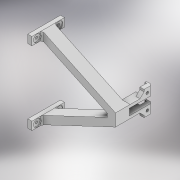
# Autodesk Inventor part: LickModule_temp
Saved by Autodesk Inventor 2020 (Build 240168000, 168)
## iProperties
Created: 2020-01-13
Part Number: LickModule_temp
Material: 일반
Document SubType Name: Modeling
Designer: Knowblesse
Density: 1 g/cm^3
Appearance: 기본값
Author: Knowblesse
## iProperties of the stored document _3D 인쇄.ipt
Created: 2021-10-22
Part Number: _3D 인쇄
Material: 일반
Document SubType Name: Modeling
Designer: Knowblesse
Density: 1 g/cm^3
Appearance: 기본값
Author: Knowblesse
Autodesk Inventor part; units mm, degrees
ref_plane "YZ Plane" through (0, 0, 0) normal (1, 0, 0) x (0, 1, 0)
ref_plane "XZ Plane" through (0, 0, 0) normal (0, 1, 0) x (-1, 0, 0)
ref_plane "XY Plane" through (0, 0, 0) normal (0, 0, 1) x (1, 0, 0)
sketch "스케치1" plane through (0, 0, 0) normal (0, 0, 1) x (1, 0, 0)
  line L0 (0, -40) -> (0, -50)
  line L1 (0, -50) -> (90, -7.5)
  line L2 (90, -7.5) -> (90, 7.5)
  line L3 (90, 7.5) -> (0, 50)
  line L4 (0, 50) -> (0, 40)
  line L5 (0, 40) -> (80, 2.2222)
  line L6 (80, 2.2222) -> (80, -2.2222)
  line L7 (80, -2.2222) -> (0, -40)
  point P0 (0, 0)
  point P1 (80, 0)
  point P2 (90, 0)
  point P3 (0, 45)
  dimension "d0" = 10
  dimension "d1" = 10
  dimension "d3" = 10
  dimension "d4" = 80
  dimension "d7" = 15
  dimension "d24" = 90
  constraints: 16 end point, 4 parallel, 3 midpoint, 2 horizontal alignment, 2 point on line, 1 vertical, 1 vertical alignment
  measures "d0" distance of L0.start L0.end
  measures "d1" distance of L3.end L4.end
  measures "d3" distance between parallel lines of L6 L2
  measures "d4" distance of L0.start L4.end
  measures "d7" distance of L1.end L2.end
  measures "d24" distance from line of point (0, 0) L2
extrude "돌출1" add sketch "스케치1" along normal blind 15
sketch "스케치2" plane through (0, 0, 0) normal (0, 0, -1) x (-1, 0, 0)
  line L0 (0, 40) -> (-80, 2.2222) projected
  line L1 (0, 50) -> (0, 40) projected
  line L2 (-90, 7.5) -> (0, 50) projected
  line L3 (-90, -7.5) -> (-90, 7.5) projected
  line L4 (0, -50) -> (-90, -7.5) projected
  line L5 (0, -40) -> (0, -50) projected
  line L6 (-80, -2.2222) -> (0, -40) projected
  line L7 (-80, 2.2222) -> (-80, -2.2222) projected
  line L8 (-90, -7.5) -> (-80, -7.5)
  line L9 (-80, -7.5) -> (-80, 7.5)
  line L10 (-80, 7.5) -> (-90, 7.5)
  line L11 (-90, 7.5) -> (-90, -7.5)
  line L12 (-80, 2.2222) -> (-80, -2.2222) projected
  point P0 (0, 0)
  point P1 (-85, 7.5)
  point P2 (-80, -2.2222)
  point P3 (-80, 2.2222)
  constraints: 8 end point, 2 parallel, 1 collinear, 1 horizontal, 1 horizontal alignment, 1 midpoint, 1 perpendicular
extrude "돌출2" add sketch "스케치2" along normal blind 30 contours L7 L9 L8 L3 L10
sketch "스케치3" plane through (0, -50, 0) normal (-1, 0, 0) x (0, 0, 1)
  line L0 (0, 100) -> (0, 90) projected
  line L1 (0, 90) -> (15, 90) projected
  line L2 (15, 100) -> (15, 90) projected
  line L3 (0, 100) -> (15, 100) projected
  line L4 (0, 10) -> (0, 0) projected
  line L5 (0, 0) -> (15, 0) projected
  line L6 (15, 10) -> (15, 0) projected
  line L7 (0, 10) -> (15, 10) projected
  line L8 (27.5, 100) -> (-12.5, 100)
  line L9 (-12.5, 100) -> (-12.5, 90)
  line L10 (-12.5, 90) -> (27.5, 90)
  line L11 (27.5, 90) -> (27.5, 100)
  line L12 (27.5, 10) -> (-12.5, 10)
  line L13 (-12.5, 10) -> (-12.5, 0)
  line L14 (-12.5, 0) -> (27.5, 0)
  line L15 (27.5, 0) -> (27.5, 10)
  line L16 (0, 90) -> (15, 90) projected
  line L17 (0, 0) -> (15, 0) projected
  line L18 (0, 10) -> (15, 10) projected
  line L19 (0, 100) -> (15, 100) projected
  point P0 (0, 50)
  point P1 (7.5, 10)
  point P2 (0, 10)
  point P3 (15, 10)
  point P4 (15, 0)
  dimension "d12" = 40
  constraints: 16 end point, 5 collinear, 4 parallel, 2 horizontal, 2 midpoint, 2 perpendicular, 1 point on line
  measures "d12" distance of L8.start L8.end
extrude "돌출3" add sketch "스케치3" along normal blind 5
sketch "스케치5" plane through (0, -50, 0) normal (1, 0, 0) x (0, 0, -1)
  line L0 (-27.5, 0) -> (-27.5, 10) projected
  line L1 (-27.5, 10) -> (12.5, 10) projected
  line L2 (12.5, 10) -> (12.5, 0) projected
  line L3 (-27.5, 90) -> (-27.5, 100) projected
  line L4 (-27.5, 100) -> (12.5, 100) projected
  line L5 (12.5, 100) -> (12.5, 90) projected
  line L6 (12.5, 90) -> (-27.5, 90) projected
  line L7 (12.5, 0) -> (-27.5, 0) projected
  point P0 (0, 50)
  point P1 (-21, 5)
  point P2 (6, 5)
  point P3 (-21, 95)
  point P4 (6, 95)
  point P5 (-27.5, 5)
  point P6 (-27.5, 95)
  dimension "d25" = 6.5
  dimension "d26" = 6.5
  constraints: 4 horizontal alignment, 2 midpoint, 2 vertical alignment
  measures "d25" distance from line of L0 point (-21, 5)
  measures "d26" distance from line of point (6, 5) L2
hole "구멍2" at (0, -45, 21) at (0, -45, -6) at (0, 45, 21) at (0, 45, -6) direction (-1, 0, 0) diameter 3 end through all counterbore diameter 9 counterbore depth 1
sketch "스케치6" plane through (90, -7.5, 15) normal (1, 0, 0) x (0, 0, -1)
  line L0 (35, -7.5) -> (45, -7.5)
  line L1 (45, -7.5) -> (45, 22.5)
  line L2 (45, 22.5) -> (35, 22.5)
  line L3 (35, 22.5) -> (35, -7.5)
  line L4 (15, 15) -> (0, 15) projected
  line L5 (0, 0) -> (0, 15) projected
  line L6 (15, 0) -> (0, 0) projected
  line L7 (15, 0) -> (45, 0) projected
  line L8 (45, 15) -> (45, 0) projected
  line L9 (15, 15) -> (45, 15) projected
  line L10 (45, 15) -> (45, 0) projected
  point P0 (15, 7.5)
  point P1 (45, 7.5)
  dimension "d34" = 30
  dimension "d35" = 10
  constraints: 8 end point, 2 midpoint, 2 parallel, 1 collinear, 1 horizontal, 1 perpendicular
  measures "d34" distance between parallel lines of L2 L0
  measures "d35" distance between parallel lines of L3 L1
extrude "돌출4" add sketch "스케치6" against normal blind 5 contours L3 L7 L1 L0 | L3 L9 L1 L7 | L3 L2 L1 L9
sketch "스케치11" plane through (80, -2.2222, 15) normal (-1, 0, 0) x (0, 0, 1)
  line L0 (-15, 0) -> (0, 0) projected
  line L1 (0, 4.4444) -> (0, 0) projected
  line L2 (-15, 4.4444) -> (0, 4.4444) projected
  line L3 (-15, 9.7222) -> (-15, 4.4444) projected
  line L4 (-15, 9.7222) -> (-45, 9.7222) projected
  line L5 (-45, -5.2778) -> (-45, 9.7222) projected
  line L6 (-15, -5.2778) -> (-45, -5.2778) projected
  line L7 (-15, 0) -> (-15, -5.2778) projected
  line L8 (-15, 9.7222) -> (-35, 9.7222) projected
  line L9 (-35, 9.7222) -> (-35, 6.2222)
  line L10 (-35, 6.2222) -> (-17, 6.2222)
  line L11 (-17, 6.2222) -> (-17, -1.7778)
  line L12 (-17, -1.7778) -> (-35, -1.7778)
  line L13 (-35, -1.7778) -> (-35, -5.2778)
  point P0 (-15, 2.2222)
  dimension "d62" = 8
  dimension "d63" = 18
  constraints: 10 end point, 3 perpendicular, 1 collinear, 1 point on line, 1 vertical
  measures "d62" distance of L10.end L11.end
  measures "d63" distance between parallel lines of L11 L13
extrude "돌출8" cut sketch "스케치11" against normal up to surface (5 mm away) contours L6 L5 L4 L9 L10 L11 L12 L13
sketch "스케치14" plane through (85, -7.5, 15) normal (-1, 0, 0) x (0, 0, 1)
  line L0 (-45, 22.5) -> (-45, -7.5) projected
  line L1 (-45, -7.5) -> (-35, -7.5) projected
  line L2 (-35, -7.5) -> (-35, 0) projected
  line L3 (-35, 3.5) -> (-35, 0) projected
  line L4 (-17, 3.5) -> (-35, 3.5) projected
  line L5 (-17, 11.5) -> (-17, 3.5) projected
  line L6 (-35, 11.5) -> (-17, 11.5) projected
  line L7 (-35, 15) -> (-35, 11.5) projected
  line L8 (-35, 15) -> (-35, 22.5) projected
  line L9 (-35, 22.5) -> (-45, 22.5) projected
  line L10 (-35, 11.5) -> (-45, 11.5)
  line L11 (-45, -7.5) -> (-45, 22.5) projected
  line L12 (-35, 3.5) -> (-45, 3.5)
  point P0 (-15, 7.5)
  constraints: 4 end point, 2 perpendicular, 2 point on line
extrude "돌출10" cut sketch "스케치14" against normal up to surface (5 mm away) contours L10 L6 L5 L4 L12 L0
sketch "스케치12" plane through (85, -7.5, 15) normal (-1, 0, 0) x (0, 0, 1)
  line L0 (-45, 22.5) -> (-45, 11.5) projected
  line L1 (-45, -7.5) -> (-35, -7.5) projected
  line L2 (-35, -7.5) -> (-35, 0) projected
  line L3 (-35, 3.5) -> (-35, 0) projected
  line L4 (-35, 15) -> (-35, 11.5) projected
  line L5 (-35, 15) -> (-35, 22.5) projected
  line L6 (-35, 22.5) -> (-45, 22.5) projected
  line L7 (-43, 22.5) -> (-45, 22.5)
  line L8 (-45, 22.5) -> (-45, -7.5)
  line L9 (-45, -7.5) -> (-43, -7.5)
  line L10 (-43, -7.5) -> (-43, 22.5)
  line L11 (-35, 3.5) -> (-45, 3.5) projected
  line L12 (-45, 3.5) -> (-45, -7.5) projected
  line L13 (-45, 11.5) -> (-35, 11.5) projected
  point P0 (-15, 7.5)
  point P1 (-43, 3.5)
  point P2 (-43, 11.5)
  dimension "d66" = 2
  constraints: 8 end point, 2 parallel, 1 horizontal, 1 perpendicular
  measures "d66" distance of L1.start L9.end
extrude "돌출9" add sketch "스케치12" along normal blind 2 contours L6 L10 L13 L0 | L11 L10 L1 L8
sketch "스케치13" plane through (85, -7.5, 15) normal (-1, 0, 0) x (0, 0, 1)
  line L0 (-43, 22.5) -> (-43, 11.5) projected
  line L1 (-35, -7.5) -> (-35, 0) projected
  line L2 (-35, 15) -> (-35, 11.5) projected
  line L3 (-35, 22.5) -> (-43, 22.5) projected
  line L4 (-43, 11.5) -> (-35, 11.5) projected
  line L5 (-35, 15) -> (-35, 22.5) projected
  line L6 (-43, 3.5) -> (-43, -7.5) projected
  line L7 (-43, -7.5) -> (-35, -7.5) projected
  line L8 (-35, 3.5) -> (-35, 0) projected
  line L9 (-35, 3.5) -> (-43, 3.5) projected
  point P0 (-15, 7.5)
  point P1 (-39, 16.75)
  point P2 (-39, -1.75)
  dimension "d69" = 5.75
  dimension "d71" = 4
  constraints: 1 vertical alignment
  measures "d69" distance from line of L3 point (-39, 16.75)
  measures "d71" distance from line of point (-39, -1.75) L1
hole "구멍4" at (85, 9.25, -24) at (85, -9.25, -24) direction (1, 0, 0) diameter 3.242 depth 5 thread size "M4x0.7" class "6H" standard "ISO Metric profile"
chamfer "모따기2" distance 2 angle 45 2 edges at (90, 9.5, -30) (90, -9.5, -30)
chamfer "모따기3" distance 5 angle 45 2 edges at (87.5, 7.5, -20) (87.5, -7.5, -20)
chamfer "모따기4" distance 3 angle 45 2 edges at (85, 7.5, 0) (85, -7.5, 0)
chamfer "모따기5" distance 2 angle 45 4 edges at (0, 45, 15) (0, 45, 0) (0, -45, 0) (0, -45, 15)
